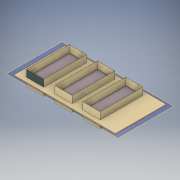
# Autodesk Inventor part: Foor
Saved by Autodesk Inventor 2018 (Build 220112000, 112)
## iProperties
Created: 2019-05-10
Part Number: Foor
Material: Generic
Document SubType Name: Modeling
Designer: 10043883
Density: 1 g/cm^3
Appearance: Wheat
Author: 10043883
Autodesk Inventor part; units mm, degrees
ref_plane "YZ Plane" through (0, 0, 0) normal (1, 0, 0) x (0, 1, 0)
ref_plane "XZ Plane" through (0, 0, 0) normal (0, 1, 0) x (-1, 0, 0)
ref_plane "XY Plane" through (0, 0, 0) normal (0, 0, 1) x (1, 0, 0)
sketch "Sketch1" plane through (0, 0, 0) normal (0, 1, 0) x (-1, 0, 0)
  line L0 (3048, 1524) -> (-3048, 1524)
  line L1 (-3048, 1524) -> (-3048, -1524)
  line L2 (-3048, -1524) -> (3048, -1524)
  line L3 (3048, -1524) -> (3048, 1524)
  line L4 (3048, 1524) -> (-3048, -1524) construction
  line L5 (-3048, 1524) -> (3048, -1524) construction
  point P0 (0, 0)
  dimension "d0" = 6096
  dimension "d1" = 3048
  constraints: 12 end point, 2 midpoint, 2 parallel, 1 horizontal, 1 perpendicular
  measures "d0" distance of L2.end L1.end
  measures "d1" distance of L1.end L0.end
extrude "Extrusion1" add sketch "Sketch1" along normal blind 254
pattern_linear "Rectangular Pattern1" count 6 spacing 6096 along (1, 0, 0) count 6 spacing 3048 along (0, 0, -1) of "Extrusion1"
sketch "Sketch2" plane through (0, 254, 0) normal (0, 1, 0) x (1, 0, 0)
  line L0 (0, 0) -> (6229.0325, 0)
  line L1 (6229.0325, 0) -> (6229.0325, 15403.294)
  line L2 (6229.0325, 15403.294) -> (0, 15403.294)
  line L3 (0, 15403.294) -> (0, 0)
  constraints: 8 end point, 2 parallel, 1 horizontal, 1 perpendicular
extrude "Extrusion2" add sketch "Sketch2" along normal blind 2540
pattern_linear "Rectangular Pattern2" count 3 spacing 10160 along (1, 0, 0) of "Extrusion2"
shell "Shell1" thickness 2.54 removed faces 3 at (22396.3442, 2794, -10268.8627) at (12236.3442, 2794, -10268.8627) at (2076.3442, 2794, -10268.8627)
ref_plane "Work Plane1" through (0, 125.73, 0) normal (0, -1, 0) x (1, 0, 0)
mirror "Mirror1" about plane through (0, 125.73, 0) normal (0, -1, 0) of "Extrusion2", "Rectangular Pattern2"
body "Solid1"
